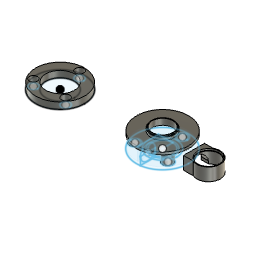
uav-base (Autodesk Fusion 360 design; units mm, degrees)
Autodesk Fusion 360 part; units mm, degrees
sketch "Sketch1" plane through (0, 0, 0) normal (0, 0, 1) x (1, 0, 0)
  circle A0 centre (0, 0) radius 27.94
  circle A1 centre (0, 0) radius 47.625
  circle A2 centre (0, 38) radius 7.94
  circle A3 centre (31.4736, -20.6814) radius 7.94
  circle A4 centre (-31.5264, -20.6814) radius 7.94
  dimension "d1" = 55.88
  dimension "d2" = 95.25
  dimension "d3" = 15.88
  dimension "d4" = 15.88
  dimension "d5" = 15.88
  constraint coincident A0.centre A1.centre
  measures "d1" diameter of A0
  measures "d2" diameter of A1
  measures "d3" diameter of A2
  measures "d4" diameter of A3
  measures "d5" diameter of A4
extrude "Extrude1" add sketch "Sketch1" along normal blind 12.7 makes body 1
sketch "Sketch2" plane through (0, 0, 0) normal (0, 0, 1) x (1, 0, 0)
  circle A0 centre (200, 0) radius 27.94
  circle A1 centre (200, 0) radius 50.8
  circle A2 centre (200, 39) radius 7.94
  circle A3 centre (200, 39) radius 10
  dimension "d8" = 55.88
  dimension "d9" = 101.6
  dimension "d10" = 15.88
  constraint concentric A0 A1
  constraint concentric A2 A3
  measures "d8" diameter of A0
  measures "d9" diameter of A1
  measures "d10" diameter of A2
extrude "Extrude2" add sketch "Sketch2" along normal blind 25.4 separate body contours A3 makes body 2
extrude "Extrude3" add sketch "Sketch2" along normal blind 5 contours A1 bodies 2
sketch "Sketch3" plane through (0, 0, 5) normal (0, 0, 1) x (-1, 0, 0)
  circle A0 centre (-200, 0) radius 27.94
  circle A1 centre (-200, -39) radius 10
  circle A2 centre (-200, 0) radius 50.8
  circle A3 centre (-232.6317, 21.9981) radius 7.94
  circle A4 centre (-232.6317, 21.9981) radius 10.0189
  circle A5 centre (-168.1475, 21.9981) radius 7.94
  circle A6 centre (-168.1475, 21.9981) radius 10
  dimension "d15" = 15.88
  dimension "d16" = 15.88
  dimension "d17" = 20
  constraint concentric A3 A4
  constraint concentric A5 A6
  measures "d15" diameter of A3
  measures "d16" diameter of A5
  measures "d17" diameter of A6
extrude "Extrude4" add sketch "Sketch3" along normal blind 20.4 contours A4 | A6 bodies 2
extrude "Extrude5" add sketch "Sketch2" along normal blind 5 contours A2 bodies 2
sketch "Sketch4" plane through (0, 0, 0) normal (0, 0, 1) x (1, 0, 0)
  circle A0 centre (200, 0) radius 22.86
  circle A1 centre (200, 0) radius 0.7
  dimension "d24" = 45.72
  dimension "d25" = 1.4
  constraint concentric A0 A1
  measures "d24" diameter of A0
  measures "d25" diameter of A1
sketch "Sketch5" plane through (0, 0, 0) normal (0, 0, 1) x (1, 0, 0)
  circle A0 centre (200, 0) radius 20
extrude "Extrude6" add sketch "Sketch2" along normal blind 5 contours A0 bodies 2
extrude "Extrude7" add sketch "Sketch4" against normal blind 15 bodies 2
extrude "Extrude8" cut sketch "Sketch5" along normal blind -20 and the other way blind -5 bodies 2
sketch "Sketch6" plane through (0, 0, 0) normal (0, 0, 1) x (1, 0, 0)
  line L0 (200, 20) -> (171.9511, 20)
  line L1 (171.9511, 20) -> (171.9511, -21)
  line L2 (171.9511, -21) -> (200, -21)
  line L3 (200, -21) -> (200, 20)
  dimension "d34" = 41
  constraint horizontal L0
  constraint vertical L1
  constraint horizontal L2
  constraint vertical L3
  measures "d34" distance of L0.start L2.end
extrude "Extrude9" add sketch "Sketch6" against normal blind 15 bodies 2
extrude "Extrude10" cut sketch "Sketch5" against normal blind 20 bodies 2
extrude "Extrude11" add 1 faces at (174.6341, -0.3333, -15) along direction (0, 0, -1) blind 10 on bodies 2 bodies 2
sketch "Sketch7" plane through (171.9511, 0, 0) normal (-1, 0, 0) x (0, -1, 0)
  line L0 (21, 0) -> (-20, 0)
  line L1 (-20, 0) -> (-20, -25)
  line L2 (-20, -25) -> (21, -25)
  line L3 (21, -25) -> (21, 0)
  circle A0 centre (0.5, -19.9354) radius 14.5
  line L4 (-13.9988, -19.746) -> (15.0012, -19.746)
  line L5 (15.0012, -19.746) -> (15.0012, -35)
  line L6 (15.0012, -35) -> (-13.9988, -35)
  line L7 (-13.9988, -35) -> (-13.9988, -19.746)
  dimension "d41" = 29
  dimension "d42" = 29
  constraint horizontal L4
  constraint vertical L5
  constraint horizontal L6
  constraint vertical L7
  constraint coincident A0 L4.start
  measures "d41" diameter of A0
  measures "d42" distance of L4.start L4.end
extrude "Extrude12" cut sketch "Sketch7" against normal blind 26 contours L2 A0 L4 | L2 A0 L5 L6 L7 | L2 A0 L5 | A0 L4 | L2 A0 L7 | L2 A0 | A0 L4 L5 bodies 2
sketch "Sketch8" plane through (171.9511, -0.5, -12.5) normal (-1, 0, 0) x (0, -1, 0)
  circle A0 centre (-17.5, -7) radius 1
  circle A1 centre (17.5, -7) radius 1
extrude "Extrude13" cut sketch "Sketch8" against normal blind 11 bodies 2
ref_plane "WorkPlane1" through (200, 0, 0) normal (0, 0, 1) x (1, 0, 0)
split "Split1" by plane through (200, 0, 0) normal (0, 0, 1) bodies 2 makes body 3 at (164.3674, -0.3333, 0)
move_body "Move1" bodies 2 to x (1, 0, 0) y (0, 1, 0) z (0, 0, 1) at (0, 0, -20)
extrude "Extrude14" add sketch "Sketch4" against normal blind 5 bodies 3
extrude "Extrude15" cut sketch "Sketch5" against normal blind 5 bodies 3
sketch "Sketch9" plane through (0, 0, -5) normal (0, 0, -1) x (1, 0, 0)
  circle A0 centre (200, 0) radius 20
  circle A1 centre (200, 0) radius 22.86
  circle A2 centre (200, 0) radius 21.3933
  constraint concentric A0 A2
sketch "Sketch10" plane through (0, 0, -5) normal (0, 0, -1) x (1, 0, 0)
extrude "Extrude16" add sketch "Sketch9" along normal blind 2 contours A2 bodies 3
sketch "Sketch11" plane through (0, 0, -20) normal (0, 0, 1) x (-1, 0, 0)
  line L0 (-171.9511, -20) -> (-171.9511, 21)
  line L1 (-171.9511, 21) -> (-190.9679, 21)
  arc A0 (-190.9679, 21) -> (-188.9284, -20) centre (-200, 0) ccw
  line L2 (-188.9284, -20) -> (-171.9511, -20)
  circle A1 centre (-200, 0) radius 20
  circle A2 centre (-200, 0) radius 21.395
  dimension "d54" = 42.79
  constraint concentric A0 A2
  measures "d54" diameter of A2
extrude "Extrude17" cut sketch "Sketch11" against normal blind 3 contours A2 bodies 2
move_body "Move2" bodies 2 to x (1, 0, 0) y (0, 1, 0) z (0, 0, 1) at (90, 0, 50)
move_body "Move3" bodies 3 to x (-1, 0, 0) y (0, 1, 0) z (0, 0, -1) at (400.2633, 0, 30.4)
equation "d9 = 4\""
equation "d11 = 1\""
